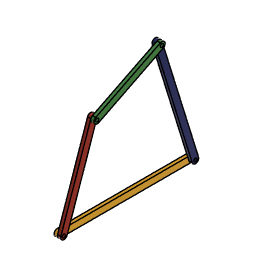
Double Rocker v1 (Autodesk Fusion 360 design; units mm, degrees)
Autodesk Fusion 360 part; units mm, degrees
sketch "Sketch1" plane through (0, 0, 0) normal (1, 0, 0) x (0, 1, 0)
  line L0 (100, -5) -> (-100, -5)
  line L1 (-100, 5) -> (100, 5)
  line L2 (100, -5) -> (-100, 5) construction
  line L3 (-100, -5) -> (100, 5) construction
  arc A0 (-99.5012, 4.9751) -> (-99.5012, -4.9751) centre (-100, 0) ccw
  arc A1 (99.5012, -4.9751) -> (99.5012, 4.9751) centre (100, 0) ccw
  circle A2 centre (-100, 0) radius 2.5
  circle A3 centre (100, 0) radius 2.5
  dimension "d1" = 5
  dimension "d2" = 5
  constraint horizontal L0
  constraint parallel L0 L1
  constraint coincident L2 origin
  constraint coincident L3 origin
  constraint coincident L0.end A0
  constraint tangent L0 A0
  constraint coincident L1.start A0
  constraint coincident L0.start A1
  constraint tangent L0 A1
  constraint coincident L1.end A1
  constraint coincident L3 A0.end
  constraint coincident L2 A0.start
  constraint coincident L3 A1.end
  constraint coincident L2 A1.start
  constraint concentric A0 A2
  constraint concentric A1 A3
  measures "d1" diameter of A2
  measures "d2" diameter of A3
extrude "Extrude1" add sketch "Sketch1" along normal blind 5 makes body 1
sketch "Sketch2" plane through (0, 0, 0) normal (1, 0, 0) x (0, 1, 0)
  line L0 (70, 5) -> (-70, 5)
  line L1 (-70, -5) -> (70, -5)
  line L2 (70, 5) -> (-70, -5) construction
  line L3 (-70, 5) -> (70, -5) construction
  arc A0 (-69.2893, 4.9492) -> (-69.2893, -4.9492) centre (-70, 0) ccw
  arc A1 (69.2893, -4.9492) -> (69.2893, 4.9492) centre (70, 0) ccw
  circle A2 centre (-70, 0) radius 2.5
  circle A3 centre (70, 0) radius 2.5
  dimension "d5" = 140
  dimension "d6" = 10
  dimension "d7" = 5
  dimension "d8" = 5
  constraint horizontal L0
  constraint parallel L0 L1
  constraint coincident L2 origin
  constraint coincident L3 origin
  constraint coincident L1.start A0
  constraint tangent L1 A0
  constraint coincident L0.end A0
  constraint coincident L1.end A1
  constraint tangent L1 A1
  constraint coincident L0.start A1
  constraint coincident L2 A0.end
  constraint coincident L3 A0.start
  constraint coincident L2 A1.end
  constraint coincident L3 A1.start
  constraint concentric A0 A2
  constraint concentric A1 A3
  measures "d5" distance of L1.start L1.end
  measures "d6" distance of L0.end L1.start
  measures "d7" diameter of A2
  measures "d8" diameter of A3
extrude "Extrude2" add sketch "Sketch2" along normal blind 5 separate body makes body 2
sketch "Sketch3" plane through (0, 0, 0) normal (1, 0, 0) x (0, 1, 0)
  line L0 (55, -5) -> (-55, -5)
  line L1 (-55, 5) -> (55, 5)
  line L2 (55, -5) -> (-55, 5) construction
  line L3 (-55, -5) -> (55, 5) construction
  arc A0 (-54.0984, 4.918) -> (-54.0984, -4.918) centre (-55, 0) ccw
  arc A1 (54.0984, -4.918) -> (54.0984, 4.918) centre (55, 0) ccw
  circle A2 centre (55, 0) radius 2.5
  circle A3 centre (-55, 0) radius 2.5
  dimension "d11" = 110
  dimension "d12" = 5
  dimension "d13" = 5
  constraint horizontal L0
  constraint parallel L0 L1
  constraint coincident L2 origin
  constraint coincident L3 origin
  constraint coincident L0.end A0
  constraint tangent L0 A0
  constraint coincident L1.start A0
  constraint coincident L0.start A1
  constraint tangent L0 A1
  constraint coincident L1.end A1
  constraint coincident L3 A0.end
  constraint coincident L2 A0.start
  constraint coincident L3 A1.end
  constraint coincident L2 A1.start
  constraint concentric A1 A2
  constraint concentric A0 A3
  measures "d11" distance of L1.start L1.end
  measures "d12" diameter of A2
  measures "d13" diameter of A3
extrude "Extrude3" add sketch "Sketch3" along normal blind 5 separate body makes body 3
sketch "Sketch4" plane through (0, 0, 0) normal (1, 0, 0) x (0, 1, 0)
  line L0 (95, -5) -> (-95, -5)
  line L1 (-95, 5) -> (95, 5)
  line L2 (95, -5) -> (-95, 5) construction
  line L3 (-95, -5) -> (95, 5) construction
  arc A0 (-94.4751, 4.9724) -> (-94.4751, -4.9724) centre (-95, 0) ccw
  arc A1 (94.4751, -4.9724) -> (94.4751, 4.9724) centre (95, 0) ccw
  circle A2 centre (-95, 0) radius 2.5
  circle A3 centre (95, 0) radius 2.5
  dimension "d16" = 190
  dimension "d17" = 5
  dimension "d18" = 5
  constraint horizontal L0
  constraint parallel L0 L1
  constraint coincident L2 origin
  constraint coincident L3 origin
  constraint coincident L0.end A0
  constraint tangent L0 A0
  constraint coincident L1.start A0
  constraint coincident L0.start A1
  constraint tangent L0 A1
  constraint coincident L1.end A1
  constraint coincident L3 A0.end
  constraint coincident L2 A0.start
  constraint coincident L3 A1.end
  constraint coincident L2 A1.start
  constraint concentric A0 A2
  constraint concentric A1 A3
  measures "d16" distance of L1.start L1.end
  measures "d17" diameter of A2
  measures "d18" diameter of A3
extrude "Extrude4" add sketch "Sketch4" along normal blind 5 separate body makes body 4
copy_body "Body->Comp1" bodies 4 removing the originals makes body 5 in component "L4(190mm)"
copy_body "Body->Comp2" bodies 3 removing the originals makes body 6 in component "L3(110mm)"
copy_body "Body->Comp3" bodies 2 removing the originals makes body 7 in component "L2(140mm)"
copy_body "Body->Comp4" bodies 1 removing the originals makes body 8 in component "L1(200mm)"
component "L4(190mm)" placed x (1, 0, 0) y (0, 0.584211, -0.811602) z (0, 0.811602, 0.584211) at (5, 44.5, 77.1022)
component "L3(110mm)" placed x (1, 0, 0) y (0, 0.989862, 0.142034) z (0, -0.142034, 0.989862) at (10, -65.4424, 146.3925)
component "L2(140mm)" placed x (1, 0, 0) y (0, -0.142034, 0.989862) z (0, -0.989862, -0.142034) at (5, -109.9424, 69.2903)
component "L1(200mm)" placed x (1, 0, 0) y (0, 1, 0) z (0, 0, 1) at (0, 0, 0)
named bodies: "L1(200mm)", "L2(140mm)", "L3(110mm)", "L4(190mm)"
